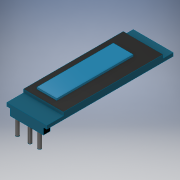
# Autodesk Inventor part: OLED_128x32
Saved by Autodesk Inventor 2017.2 (Build 212223000, 223)
## iProperties
Created: 2017-02-28
Part Number: OLED_128x32
Material: Generic
Document SubType Name: Modeling
Designer: prosp
Density: 1 g/cm^3
Appearance: Sky Blue Dark
Author: prosp
Autodesk Inventor part; units mm, degrees
ref_plane "YZ Plane" through (0, 0, 0) normal (1, 0, 0) x (0, 1, 0)
ref_plane "XZ Plane" through (0, 0, 0) normal (0, 1, 0) x (-1, 0, 0)
ref_plane "XY Plane" through (0, 0, 0) normal (0, 0, 1) x (1, 0, 0)
sketch "Sketch1" plane through (0, 0, 0) normal (0, 1, 0) x (-1, 0, 0)
  line L0 (6, 19) -> (6, -19)
  line L1 (6, -19) -> (-6, -19)
  line L2 (-6, -19) -> (-6, 19)
  line L3 (-6, 19) -> (6, 19)
  line L4 (6, 19) -> (-6, -19) construction
  line L5 (6, -19) -> (-6, 19) construction
  point P0 (0, 0)
  dimension "d0" = 38
  dimension "d1" = 12
  constraints: 12 end point, 2 midpoint, 2 parallel, 1 perpendicular, 1 vertical
  measures "d0" distance of L0.start L0.end
  measures "d1" distance of L0.end L1.end
extrude "Extrusion1" add sketch "Sketch1" along normal blind 1
sketch "Sketch2" plane through (0, 1, 0) normal (0, 1, 0) x (1, 0, 0)
  point P0 (0, 0)
sketch "Sketch3" plane through (0, 1, 0) normal (0, 1, 0) x (1, 0, 0)
  line L0 (-6, -14) -> (-6, 16)
  line L1 (-6, 16) -> (6, 16)
  line L2 (6, 16) -> (6, -14)
  line L3 (6, -14) -> (-6, -14)
  line L4 (-6, -14) -> (6, 16) construction
  line L5 (-6, 16) -> (6, -14) construction
  line L6 (-6, -19) -> (6, -19) projected
  line L7 (-6, 19) -> (-6, -19) projected
  line L8 (-6, 16) -> (-6, 19)
  dimension "d4" = 30
  dimension "d5" = 12
  constraints: 14 end point, 2 parallel, 1 collinear, 1 perpendicular, 1 vertical
  measures "d4" distance of L0.start L0.end
  measures "d5" distance of L0.end L1.end
extrude "Extrusion2" add sketch "Sketch3" along normal blind 1
sketch "Sketch4" plane through (0, 2, 0) normal (0, 1, 0) x (1, 0, 0)
  point P0 (0, 0)
sketch "Sketch5" plane through (0, 2, 0) normal (0, 1, 0) x (1, 0, 0)
  point P0 (0, 0)
sketch "Sketch6" plane through (0, 0, 0) normal (0, -1, 0) x (1, 0, 0)
  line L0 (-6, 19) -> (6, 19) projected
  line L1 (0, 19) -> (5, 19)
  line L2 (-5, 17) -> (-5, 19)
  line L3 (-5, 19) -> (5, 19)
  line L4 (5, 19) -> (5, 17)
  line L5 (5, 17) -> (-5, 17)
  point P0 (0, 0)
  dimension "d11" = 5
  dimension "d12" = 2
  dimension "d13" = 5
  constraints: 10 end point, 2 parallel, 2 point on line, 1 perpendicular
  measures "d11" distance of L1.start L2.end
  measures "d12" distance of L2.end L2.start
  measures "d13" distance of L1.start L1.end
extrude "Extrusion3" add sketch "Sketch6" along normal blind 2
sketch "Sketch7" plane through (0, -2, 0) normal (0, -1, 0) x (1, 0, 0)
  circle A0 centre (0, 18.0182) radius 0.5
  circle A1 centre (-3.7835, 18) radius 0.5
  circle A2 centre (2.8577, 18) radius 0.5
  point P0 (0, 0)
  dimension "d16" = 1
  dimension "d17" = 1
  dimension "d18" = 1
  constraints: 3 centre point
  measures "d16" diameter of A0
  measures "d17" diameter of A1
  measures "d18" diameter of A2
extrude "Extrusion4" add sketch "Sketch7" along normal blind 5
sketch "Sketch8" plane through (0, 2, 0) normal (0, 1, 0) x (1, 0, 0)
  line L0 (-6, -14) -> (6, -14) projected
  line L1 (-4, -12) -> (-4, 11)
  line L2 (-4, 11) -> (2, 11)
  line L3 (2, 11) -> (2, -12)
  line L4 (2, -12) -> (-4, -12)
  point P0 (0, 0)
  dimension "d31" = 23
  dimension "d32" = 6
  constraints: 8 end point, 3 perpendicular, 1 vertical
  measures "d31" distance of L1.start L1.end
  measures "d32" distance of L1.end L2.end
extrude "Extrusion5" add sketch "Sketch8" along normal blind 0.5
body "Solid1"
